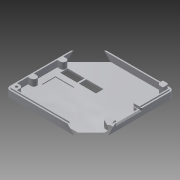
# Autodesk Inventor part: LCDDerivativeBottom1
Saved by Autodesk Inventor 2015 SP1 (Build 190203100, 203)
## iProperties
Created: 2015-04-16
Part Number: LCDDerivativeBottom1
Material: ABS Plastic
Document SubType Name: Modeling
Designer: Jack
Density: 1.06 g/cm^3
Appearance: Smooth - White
Author: Jack
Autodesk Inventor part; units mm, degrees
ref_plane "YZ Plane" through (0, 0, 0) normal (1, 0, 0) x (0, 1, 0)
ref_plane "XZ Plane" through (0, 0, 0) normal (0, 1, 0) x (-1, 0, 0)
ref_plane "XY Plane" through (0, 0, 0) normal (0, 0, 1) x (1, 0, 0)
sketch "Sketch1" plane through (0, 0, 0) normal (0, 0, 1) x (1, 0, 0)
  line L0 (0, 0) -> (-100, 0)
  line L1 (-100, 0) -> (-100, 97)
  line L2 (-100, 97) -> (0, 97)
  line L3 (0, 97) -> (0, 0)
  dimension "d0" = 100
  dimension "d1" = 97
  constraints: 8 end point, 2 parallel, 1 horizontal, 1 perpendicular
  measures "d0" distance of L1.end L2.end
  measures "d1" distance of L0.end L1.end
extrude "Extrusion1" add sketch "Sketch1" along normal blind 2
sketch "Sketch2" plane through (0, 0, 2) normal (0, 0, 1) x (1, 0, 0)
  line L0 (-100, 0) -> (0, 0) projected
  line L1 (0, 0) -> (0, 97) projected
  line L2 (0, 97) -> (-100, 97) projected
  line L3 (-100, 97) -> (-100, 0) projected
  line L4 (-98.4, 95.4) -> (-1.6, 95.4)
  line L5 (-1.6, 95.4) -> (-1.6, 1.6)
  line L6 (-1.6, 1.6) -> (-98.4, 1.6)
  line L7 (-98.4, 1.6) -> (-98.4, 95.4)
  dimension "d4" = 1.6
  constraints: 8 end point, 3 other
  measures "d4" distance between parallel lines of L2 L4
extrude "Extrusion2" add sketch "Sketch2" along normal blind 6
sketch "Sketch3" plane through (0, 0, 2) normal (0, 0, 1) x (1, 0, 0)
  line L0 (-1.6, 1.6) -> (-1.6, 95.4) projected
  line L1 (-1.6, 95.4) -> (-98.4, 95.4) projected
  line L2 (-98.4, 95.4) -> (-98.4, 1.6) projected
  line L3 (-98.4, 1.6) -> (-1.6, 1.6) projected
  line L4 (-97, 94) -> (-3, 94)
  line L5 (-3, 94) -> (-3, 3)
  line L6 (-3, 3) -> (-97, 3)
  line L7 (-97, 3) -> (-97, 94)
  point P0 (0, 0)
  dimension "d7" = 1.4
  constraints: 8 end point, 3 other
  measures "d7" distance between parallel lines of L1 L4
extrude "Extrusion3" add sketch "Sketch3" along normal blind 7.5
fillet "Fillet1" radius 4.7 4 edges at (-100, 0, 4) (0, 0, 4) (0, 97, 4) (-100, 97, 4)
sketch "Sketch10" plane through (0, 0, 2) normal (0, 0, 1) x (1, 0, 0)
  line L0 (-3, 3) -> (-3, 94) projected
  line L1 (-3, 94) -> (-97, 94) projected
  line L2 (-97, 94) -> (-97, 3) projected
  line L3 (-97, 3) -> (-3, 3) projected
  arc A0 (-10, 90.75) -> (-6.25, 87) centre (-6.25, 90.75) ccw
  arc A1 (-93.75, 87) -> (-90, 90.75) centre (-93.75, 90.75) ccw
  arc A2 (-90, 6.25) -> (-93.75, 10) centre (-93.75, 6.25) ccw
  arc A3 (-6.25, 10) -> (-10, 6.25) centre (-6.25, 6.25) ccw
  line L4 (-93.75, 10) -> (-97, 10)
  line L5 (-90, 6.25) -> (-90, 3)
  line L6 (-10, 6.25) -> (-10, 3)
  line L7 (-6.25, 10) -> (-3, 10)
  line L8 (-1.6, 1.6) -> (-1.6, 95.4) projected
  line L9 (-6.25, 87) -> (-3, 87)
  line L10 (-10, 90.75) -> (-10, 94)
  line L11 (-90, 90.75) -> (-90, 94)
  line L12 (-93.75, 87) -> (-97, 87)
  point P0 (0, 0)
  point P1 (-1.6, 4.7)
  point P2 (-1.6, 92.3)
  dimension "d57" = 3.25
  dimension "d58" = 3.25
  dimension "d59" = 3.25
  dimension "d60" = 3.25
  dimension "d61" = 7
  constraints: 16 end point, 15 point on line, 8 point on circle, 5 tangent, 4 centre point, 4 coincident, 4 perpendicular, 3 equal radius, 2 horizontal alignment, 2 vertical alignment
  measures "d57" distance from line of L3 point (-93.75, 6.25)
  measures "d58" distance from line of L2 point (-93.75, 6.25)
  measures "d59" distance from line of L0 point (-6.25, 90.75)
  measures "d60" distance from line of L1 point (-6.25, 90.75)
  measures "d61" distance between parallel lines of L1 L12
extrude "Extrusion7" add sketch "Sketch10" along normal blind 7.5 contours L3 L6 A3 L7 L0 | L9 A0 L10 L1 L0 | L3 L2 L4 A2 L5 | L11 A1 L12 L2 L1
sketch "Sketch12" plane through (0, 0, 2) normal (0, 0, 1) x (1, 0, 0)
  line L0 (-97, 87) -> (-97, 10) projected
  arc A0 (-90, 6.25) -> (-93.75, 10) centre (-93.75, 6.25) ccw projected
  arc A1 (-6.25, 10) -> (-10, 6.25) centre (-6.25, 6.25) ccw projected
  line L1 (-3, 10) -> (-3, 87) projected
  arc A2 (-93.75, 22.75) -> (-93.75, 29.75) centre (-93.75, 26.25) ccw
  arc A3 (-6.25, 29.75) -> (-6.25, 22.75) centre (-6.25, 26.25) ccw
  line L2 (-93.75, 29.75) -> (-97, 29.75)
  line L3 (-93.75, 22.75) -> (-97, 22.75)
  line L4 (-6.25, 22.75) -> (-3, 22.75)
  line L5 (-3, 94) -> (-3, 3) projected
  line L6 (-6.25, 29.75) -> (-3, 29.75)
  arc A4 (-93.75, 57.25) -> (-93.75, 64.25) centre (-93.75, 60.75) ccw
  arc A5 (-6.25, 64.25) -> (-6.25, 57.25) centre (-6.25, 60.75) ccw
  line L7 (-93.75, 64.25) -> (-97, 64.25)
  line L8 (-93.75, 57.25) -> (-97, 57.25)
  line L9 (-97, 10) -> (-97, 87) projected
  line L10 (-6.25, 64.25) -> (-3, 64.25)
  line L11 (-6.25, 57.25) -> (-3, 57.25)
  line L12 (-97, 64.25) -> (-97, 57.25)
  point P0 (0, 0)
  dimension "d71" = 20
  dimension "d72" = 7
  dimension "d148" = 7
  dimension "d149" = 34.5
  constraints: 18 end point, 10 point on line, 8 point on circle, 7 tangent, 5 perpendicular, 4 centre point, 4 coincident, 4 vertical alignment, 2 equal radius, 2 horizontal alignment, 1 collinear, 1 horizontal, 1 parallel
  measures "d71" distance of A0.centre point (-93.75, 26.25)
  measures "d72" diameter of A2
  measures "d148" diameter of A5
  measures "d149" distance of point (-93.75, 26.25) point (-93.75, 60.75)
extrude "Extrusion8" add sketch "Sketch12" along normal up to surface (7.5 mm away)
sketch "Sketch15" plane through (0, 0, 0) normal (0, 0, -1) x (-1, 0, 0)
  arc A0 (90, 90.75) -> (93.75, 87) centre (93.75, 90.75) ccw projected
  arc A1 (93.75, 29.75) -> (93.75, 22.75) centre (93.75, 26.25) ccw projected
  arc A2 (93.75, 10) -> (90, 6.25) centre (93.75, 6.25) ccw projected
  arc A3 (6.25, 87) -> (10, 90.75) centre (6.25, 90.75) ccw projected
  arc A4 (6.25, 22.75) -> (6.25, 29.75) centre (6.25, 26.25) ccw projected
  arc A5 (10, 6.25) -> (6.25, 10) centre (6.25, 6.25) ccw projected
  point P0 (0, 0)
hole "Hole4" at (-6.25, 90.75, 0) at (-93.75, 90.75, 0) at (-6.25, 6.25, 0) at (-93.75, 6.25, 0) direction (0, 0, 1) diameter 3.5 end up to face face through (-63.3333, 94.9333, 9.5) facing (0, 0, 1) counterbore diameter 5.8 counterbore depth 4.2
fillet "Fillet4" radius 3.1 4 edges at (-98.4, 1.6, 8.75) (-1.6, 1.6, 8.75) (-1.6, 95.4, 8.75) (-98.4, 95.4, 8.75)
sketch "Sketch16" plane through (0, 0, 2) normal (0, 0, 1) x (1, 0, 0)
  line L0 (-90, 3) -> (-10, 3) projected
  line L1 (-97, 87) -> (-97, 29.75) projected
  line L2 (-67, 31) -> (-89, 31)
  line L3 (-89, 31) -> (-89, 47)
  line L4 (-89, 47) -> (-67, 47)
  line L5 (-67, 47) -> (-67, 31)
  point P0 (0, 0)
  dimension "d95" = 22
  dimension "d96" = 16
  dimension "d97" = 8
  dimension "d98" = 28
  constraints: 8 end point, 2 parallel, 1 horizontal, 1 perpendicular
  measures "d95" distance of L3.end L4.end
  measures "d96" distance of L4.end L2.start
  measures "d97" distance between parallel lines of L1 L3
  measures "d98" distance between parallel lines of L0 L2
extrude "Extrusion11" cut sketch "Sketch16" against normal blind 1
sketch "Sketch17" plane through (0, 4.7, 0) normal (1, 0, 0) x (0, 0, -1)
  line L0 (-8, 87.6) -> (0, 87.6) projected
  line L1 (0, 0) -> (-8, 0) projected
  line L2 (-9.5, 89.3) -> (-9.5, -1.7) projected
  line L3 (-9.5, 53.4) -> (-6.5, 53.4)
  line L4 (-9.5, 25.7) -> (-6.5, 25.7)
  line L5 (-6.5, 25.7) -> (-6.5, 53.4)
  point P0 (0, -4.7)
  dimension "d101" = 25.7
  dimension "d102" = 34.2
  dimension "d103" = 3
  constraints: 6 end point, 2 horizontal, 2 point on line, 1 parallel
  measures "d101" distance between parallel lines of L1 L4
  measures "d102" distance between parallel lines of L0 L3
  measures "d103" distance of L3.start L3.end
extrude "Extrusion12" cut sketch "Sketch17" against normal blind 5
chamfer "Chamfer1" distance 1.4 angle 45 3 edges at (0, 58.1, 7.25) (0, 44.25, 6.5) (0, 30.4, 7.25)
sketch "Sketch22" plane through (0, 0, 0) normal (0, 0, -1) x (-1, 0, 0)
  line L0 (95.3, 97) -> (4.7, 97) projected
  line L1 (4.7, 0) -> (95.3, 0) projected
  line L2 (100, 4.7) -> (100, 92.3) projected
  line L3 (47.9, 53.4) -> (67.9, 53.4)
  line L4 (67.9, 53.4) -> (67.9, 62.2)
  line L5 (67.9, 62.2) -> (47.9, 62.2)
  line L6 (47.9, 62.2) -> (47.9, 53.4)
  line L7 (69.9, 53.4) -> (89.9, 53.4)
  line L8 (89.9, 53.4) -> (89.9, 62.2)
  line L9 (89.9, 62.2) -> (69.9, 62.2)
  line L10 (69.9, 62.2) -> (69.9, 53.4)
  point P0 (0, 0)
  dimension "d138" = 10.1
  dimension "d139" = 34.8
  dimension "d140" = 53.4
  dimension "d141" = 30.1
  dimension "d142" = 32.1
  constraints: 16 end point, 4 parallel, 2 horizontal, 2 perpendicular, 2 point on line, 1 collinear
  measures "d138" distance between parallel lines of L2 L8
  measures "d139" distance between parallel lines of L0 L9
  measures "d140" distance between parallel lines of L1 L7
  measures "d141" distance between parallel lines of L2 L10
  measures "d142" distance between parallel lines of L2 L4
extrude "Extrusion15" cut sketch "Sketch22" against normal up to next
sketch "Sketch23" plane through (0, 0, 9.5) normal (0, 0, 1) x (1, 0, 0)
  line L0 (-97, 87) -> (-93.75, 87) projected
  arc A0 (-93.75, 87) -> (-90, 90.75) centre (-93.75, 90.75) ccw projected
  line L1 (-90, 90.75) -> (-90, 94) projected
  line L2 (-10, 94) -> (-10, 90.75) projected
  arc A1 (-10, 90.75) -> (-6.25, 87) centre (-6.25, 90.75) ccw projected
  line L3 (-6.25, 87) -> (-3, 87) projected
  line L4 (-3, 87) -> (-3, 29.75) projected
  line L5 (-97, 87) -> (-97, 94)
  line L6 (-97, 94) -> (-90, 94)
  line L7 (-10, 94) -> (-3, 94)
  line L8 (-10, 90.75) -> (-10, 94) projected
  line L9 (-3, 94) -> (-3, 87)
  point P0 (-3, 58.1)
  point P1 (0, 0)
  constraints: 8 end point, 2 perpendicular, 1 collinear, 1 vertical
extrude "Extrusion16" add sketch "Sketch23" along normal blind 4.25
fillet "Fillet6" radius 2 2 edges at (-97, 94, 11.625) (-3, 94, 11.625)
sketch "Sketch24" plane through (-5, 4.7, 0) normal (1, 0, 0) x (0, 0, -1)
  line L0 (-6.5, 52.55) -> (-9.5, 52.55) projected
  line L1 (-6.5, 53.4) -> (-6.5, 52.55) projected
  line L2 (-9.5, 53.4) -> (-6.5, 53.4) projected
  line L3 (-9.5, 52.55) -> (-9.5, 53.4) projected
  point P0 (0, -4.7)
extrude "Extrusion17" cut sketch "Sketch24" against normal blind 4.5
sketch "Sketch25" plane through (-6.25, 90.75, 9.5) normal (0, 0, -1) x (-1, 0, 0)
  circle A0 centre (0, 0) radius 1.75 projected
  circle A1 centre (87.5, 0) radius 1.75 projected
  point P0 (-6.25, -90.75)
extrude "Extrusion18" cut sketch "Sketch25" against normal up to surface (4.25 mm away)
body "Solid1"
